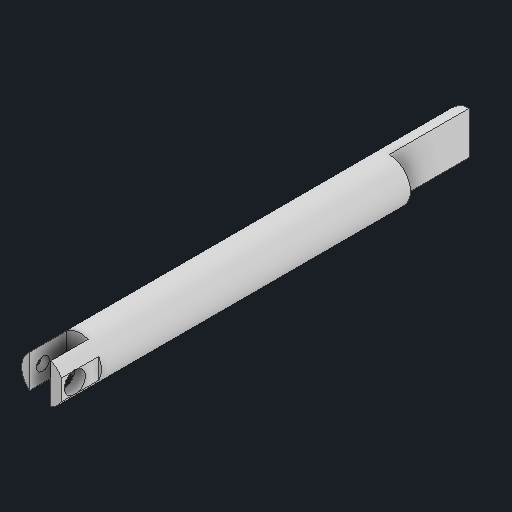
# Autodesk Inventor part: Servo_Strut_CPY_CPY
Saved by Autodesk Inventor 2023 (Build 270158000, 158)
## iProperties
Created: 2023-02-24
Part Number: Servo_Strut_CPY_CPY
Material: Generic
Document SubType Name: Modeling
Designer: roota
Density: 1 g/cm^3
Appearance: Default
Author: roota
Autodesk Inventor part; units mm, degrees
ref_plane "YZ Plane" through (0, 0, 0) normal (1, 0, 0) x (0, 1, 0)
ref_plane "XZ Plane" through (0, 0, 0) normal (0, 1, 0) x (-1, 0, 0)
ref_plane "XY Plane" through (0, 0, 0) normal (0, 0, 1) x (1, 0, 0)
sketch "Sketch1" plane through (0, 0, 0) normal (0, 0, 1) x (1, 0, 0)
  circle A0 centre (0, 0) radius 4
  dimension "d0" = 8
  constraints: 1 centre point, 1 coincident
  measures "d0" diameter of A0
extrude "Extrusion1" add sketch "Sketch1" along normal blind 80
sketch "Sketch2" plane through (0, 0, 0) normal (0, 1, 0) x (-1, 0, 0)
  line L0 (0, 0) -> (-5.3393, 0)
  line L1 (-5.3393, 0) -> (-5.3393, 15)
  line L2 (-5.3393, 15) -> (0, 15)
  line L3 (0, 15) -> (0, 0)
  line L4 (2.5, 80) -> (-1.5, 80)
  line L5 (-1.5, 80) -> (-1.5, 73)
  line L6 (-1.5, 73) -> (2.5, 73)
  line L7 (2.5, 73) -> (2.5, 80)
  line L8 (4, 80) -> (-4, 80) construction
  line L9 (-4, 80) -> (-3.5, 80)
  line L10 (-3.5, 80) -> (-3.5, 73)
  line L11 (-3.5, 73) -> (-4, 73)
  line L12 (-4, 73) -> (-4, 80)
  point P0 (-3.75, 73)
  dimension "d3" = 4
  dimension "d4" = 7
  dimension "d5" = 2.5
  dimension "d6" = 15
  dimension "d9" = 2
  constraints: 24 end point, 6 parallel, 3 horizontal, 3 perpendicular, 1 horizontal alignment, 1 midpoint, 1 point on line
  measures "d3" distance of L6.end L5.end
  measures "d4" distance of L5.end L4.end
  measures "d5" distance between parallel lines of L7 L3
  measures "d6" distance of L0.end L1.end
  measures "d9" distance between parallel lines of L5 L10
extrude "Extrusion2" cut sketch "Sketch2" along normal through all both and the other way through all
sketch "Sketch3" plane through (3.5, -1.9365, 73) normal (1, 0, 0) x (0, 0, -1)
  circle A0 centre (-4.5, 1.9365) radius 1.5
  line L0 (-7, 0) -> (-7, 3.873) projected
  point P0 (73, 1.9365)
  point P1 (-7, 1.9365)
  dimension "d10" = 3
  dimension "d11" = 2.5
  constraints: 1 centre point, 1 horizontal alignment, 1 midpoint
  measures "d10" diameter of A0
  measures "d11" distance of point (-7, 1.936) A0.centre
hole "Hole1" at (3.5, 0, 77.5) direction (-1, 0, 0) diameter 2.459 end through all counterbore diameter 4 counterbore depth 3 thread size "M3x0.5" class "6H" standard "ISO Metric profile"
body "Solid1"
